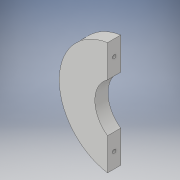
# Autodesk Inventor part: ContrapesoGrande2
Saved by Autodesk Inventor 2019 (Build 230136000, 136)
## iProperties
Created: 2019-06-29
Part Number: ContrapesoGrande2
Material: Generic
Document SubType Name: Modeling
Designer: usuario
Density: 1 g/cm^3
Appearance: Default
Author: usuario
Autodesk Inventor part; units mm, degrees
ref_plane "YZ Plane" through (0, 0, 0) normal (1, 0, 0) x (0, 1, 0)
ref_plane "XZ Plane" through (0, 0, 0) normal (0, 1, 0) x (-1, 0, 0)
ref_plane "XY Plane" through (0, 0, 0) normal (0, 0, 1) x (1, 0, 0)
sketch "Sketch1" plane through (0, 0, 0) normal (0, 0, 1) x (1, 0, 0)
  arc A0 (-5, 32.1131) -> (-5, -32.1131) centre (0, 0) ccw
  arc A1 (-5, 13.7954) -> (-5, -13.7954) centre (4.5, 0) ccw
  line L0 (-5, -13.7954) -> (-5, -32.1131)
  line L1 (-5, 13.7954) -> (-5, 32.1131)
  arc A2 (-5, 13.7954) -> (-5, -13.7954) centre (4.5, 0) ccw
  point P0 (3.7885, 24.6247)
  constraints: 6 point on circle, 4 end point, 3 centre point, 2 vertical, 1 coincident
extrude "Extrusion1" add sketch "Sketch1" along normal blind 7.5
sketch "Sketch2" plane through (-5, -32.1131, 0) normal (1, 0, 0) x (0, 0, -1)
  line L0 (0, 6.9167) -> (7.5, 6.9167)
  line L1 (0, 0) -> (0, 6.9167)
  line L2 (0, 6.9167) -> (7.5, 6.9167)
  line L3 (7.5, 26.7893) -> (7.5, 0)
  line L4 (7.5, 6.9167) -> (7.5, 0)
  line L5 (7.5, 0) -> (0, 0)
  line L6 (7.5, 0) -> (0, 0)
  circle A0 centre (-3.75, 8.7821) radius 1
  line L7 (0, 0) -> (3.0149, 2.7804)
  line L8 (4.4851, 4.1363) -> (7.5, 6.9167)
  line L9 (0, 6.9167) -> (3.0149, 4.1363)
  line L10 (4.4851, 2.7804) -> (7.5, 0)
  line L11 (0, 0) -> (0, 53.5786)
  line L12 (0, 53.5786) -> (0, 0)
  line L13 (-7.5, 32.1131) -> (0, 32.1131)
  circle A1 centre (-3.75, 55.4441) radius 1
  line L14 (0, 53.5786) -> (7.5, 53.5786)
  line L15 (7.5, 53.5786) -> (7.5, 0)
  line L16 (-7.2671, 64.2522) -> (-7.2671, 0)
  line L17 (-7.5, 64.2262) -> (-7.5, 0) projected
  line L18 (-7.5, 32.1131) -> (-4.2989, 32.1131)
  point P0 (280.32, 51.414)
  dimension "d3" = 2
  constraints: 36 end point, 3 vertical, 2 centre point, 2 collinear, 2 horizontal, 2 perpendicular, 1 midpoint, 1 symmetric about line, 1 other
  measures "d3" diameter of A0
extrude "Extrusion2" cut sketch "Sketch2" against normal blind 25.4 contours A0 | A1
body "Solid1"
